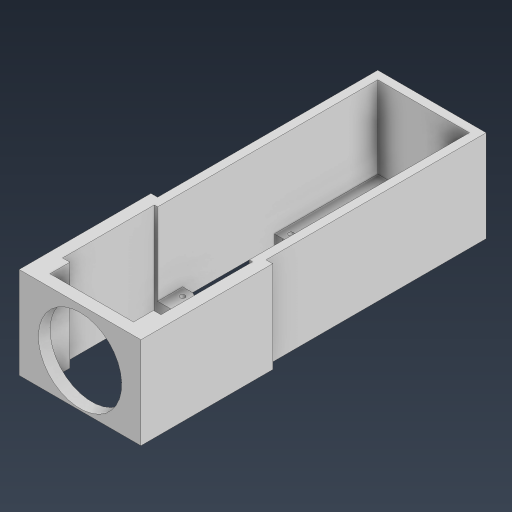
# Autodesk Inventor part: New_base_v2
Saved by Autodesk Inventor 2024 (Build 280153000, 153)
## iProperties
Created: 2025-10-20
Part Number: New_base_v2
Material: Generic
Document SubType Name: Modeling
Designer: Piter
Density: 1 g/cm^3
Appearance: Default
Author: Piter
Autodesk Inventor part; units mm, degrees
ref_plane "YZ Plane" through (0, 0, 0) normal (1, 0, 0) x (0, 1, 0)
ref_plane "XZ Plane" through (0, 0, 0) normal (0, 1, 0) x (-1, 0, 0)
ref_plane "XY Plane" through (0, 0, 0) normal (0, 0, 1) x (1, 0, 0)
sketch "Sketch1" plane through (0, 0, 0) normal (0, 1, 0) x (-1, 0, 0)
  line L0 (-22.5, 32.5) -> (22.5, 32.5) construction
  line L1 (22.5, 32.5) -> (22.5, -32.5) construction
  line L2 (22.5, -32.5) -> (-22.5, -32.5) construction
  line L3 (-22.5, -32.5) -> (-22.5, 32.5) construction
  line L4 (-22.5, 32.5) -> (22.5, -32.5) construction
  line L5 (22.5, 32.5) -> (-22.5, -32.5) construction
  circle A0 centre (22.5, 32.5) radius 1.5
  circle A1 centre (22.5, -32.5) radius 1.5
  circle A2 centre (-22.5, -32.5) radius 1.5
  circle A3 centre (-22.5, 32.5) radius 1.5
  line L6 (27.5, 30) -> (-27.5, 30)
  line L7 (-27.5, 30) -> (-27.5, 37.5)
  line L8 (-27.5, 37.5) -> (27.5, 37.5)
  line L9 (27.5, 37.5) -> (27.5, 30)
  line L10 (27.5, -30) -> (27.5, -37.5)
  line L11 (27.5, -37.5) -> (-27.5, -37.5)
  line L12 (-27.5, -37.5) -> (-27.5, -30)
  line L13 (-27.5, -30) -> (27.5, -30)
  circle A4 centre (22.5, 32.5) radius 5
  circle A5 centre (22.5, -32.5) radius 5
  circle A6 centre (-22.5, -32.5) radius 5
  circle A7 centre (-22.5, 32.5) radius 5
  line L14 (-27.5, 37.5) -> (27.5, 37.5)
  line L15 (27.5, 37.5) -> (27.5, -37.5)
  line L16 (27.5, -37.5) -> (-27.5, -37.5)
  line L17 (-27.5, -37.5) -> (-27.5, 37.5)
  line L18 (-27.5, 37.5) -> (27.5, -37.5) construction
  line L19 (27.5, 37.5) -> (-27.5, -37.5) construction
  line L20 (-32.5, 42.5) -> (32.5, 42.5)
  line L21 (32.5, 42.5) -> (32.5, -42.5)
  line L22 (32.5, -42.5) -> (-32.5, -42.5)
  line L23 (-32.5, -42.5) -> (-32.5, 42.5)
  line L24 (-32.5, 42.5) -> (32.5, -42.5) construction
  line L25 (32.5, 42.5) -> (-32.5, -42.5) construction
  line L26 (32.5, 42.5) -> (-14.872, 42.5)
  line L27 (0, 0) -> (0, -184) construction
  line L28 (-21, -47.5) -> (21, -47.5)
  line L29 (21, -47.5) -> (21, -89.5)
  line L30 (21, -89.5) -> (-21, -89.5)
  line L31 (-21, -89.5) -> (-21, -47.5)
  line L32 (-21, -47.5) -> (21, -89.5) construction
  line L33 (21, -47.5) -> (-21, -89.5) construction
  line L34 (32.5, -42.5) -> (32.5, -94.5)
  line L35 (32.5, -94.5) -> (-32.5, -94.5)
  line L36 (-32.5, -94.5) -> (-32.5, -42.5)
  line L37 (22.5, 27.5) -> (27.5, 27.5)
  line L38 (22.5, -27.5) -> (27.5, -27.5)
  line L39 (-22.5, -27.5) -> (-27.5, -27.5)
  line L40 (-22.5, 27.5) -> (-27.5, 27.5)
  line L41 (0, 0) -> (0, 113) construction
  line L42 (32.5, 42.5) -> (32.5, 97.5)
  line L43 (32.5, 97.5) -> (-32.5, 97.5)
  line L44 (-32.5, 97.5) -> (-32.5, 42.5)
  line L45 (29.5, 42.5) -> (29.5, 97.5)
  line L46 (-29.5, 97.5) -> (-29.5, 42.5)
  line L47 (32.5, 42.5) -> (36.5, 42.5)
  line L48 (36.5, 42.5) -> (36.5, 112.5)
  line L49 (36.5, 112.5) -> (-36.5, 112.5)
  line L50 (-36.5, 112.5) -> (-36.5, 42.5)
  line L51 (-36.5, 42.5) -> (-32.5, 42.5)
  line L52 (-27.5, 37.5) -> (-36.5, 37.5)
  line L53 (-36.5, 37.5) -> (-36.5, 42.5)
  line L54 (-27.5, -27.5) -> (-26.5, -27.5)
  line L55 (-26.5, -27.5) -> (-26.5, 27.5)
  line L56 (0, 112.5) -> (0, 97.5)
  line L57 (-25.05, 112.5) -> (25.05, 112.5)
  line L58 (25.05, 112.5) -> (25.05, 97.5)
  line L59 (25.05, 97.5) -> (-25.05, 97.5)
  line L60 (-25.05, 97.5) -> (-25.05, 112.5)
  line L61 (-25.05, 112.5) -> (25.05, 97.5) construction
  line L62 (25.05, 112.5) -> (-25.05, 97.5) construction
  line L63 (25.05, 109.5) -> (-25.05, 109.5)
  line L64 (36.5, 112.5) -> (-36.5, 112.5)
  line L65 (-36.5, 112.5) -> (-36.5, 116.5)
  line L66 (-36.5, 116.5) -> (36.5, 116.5)
  line L67 (36.5, 116.5) -> (36.5, 112.5)
  line L68 (36.5, 42.5) -> (36.5, 37.5)
  line L69 (36.5, 37.5) -> (32.5, 37.5)
  point P0 (0, -68.5)
  point P1 (18.1699, 30)
  point P2 (18.1699, -30)
  point P3 (-18.1699, -30)
  point P4 (-18.1699, 30)
  point P5 (-32.5, 70)
  point P6 (32.5, 0)
  point P7 (-32.5, 37.5)
  point P8 (0, 105)
  point P9 (-25.05, 97.5)
  dimension "d8" = 10
  dimension "d9" = 10
  dimension "d10" = 10
  dimension "d11" = 10
  dimension "d0" = 45
  dimension "d1" = 65
  dimension "d2" = 3
  dimension "d3" = 3
  dimension "d4" = 3
  dimension "d5" = 3
  dimension "d6" = 2.5
  dimension "d7" = 2.5
  dimension "d12" = 5
  dimension "d13" = 5
  dimension "d17" = 42
  dimension "d18" = 42
  dimension "d19" = 5
  dimension "d20" = 5
  dimension "d38" = 55
  dimension "d39" = 3
  dimension "d40" = 3
  dimension "d41" = 4
  dimension "d42" = 4
  dimension "d43" = 15
  dimension "d57" = 1
  dimension "d72" = 50.1
  dimension "d84" = 7
  dimension "d85" = 3
  constraints: 141 end point, 29 perpendicular, 22 point on line, 15 horizontal, 15 midpoint, 12 parallel, 9 vertical, 8 coincident, 4 centre point, 2 collinear, 12 other
  measures "d0" distance of L1.end L2.end
  measures "d1" distance of L0.end L1.end
  measures "d2" diameter of A0
  measures "d3" diameter of A1
  measures "d4" diameter of A2
  measures "d5" diameter of A3
  measures "d6" distance from line of A0.centre L6
  measures "d7" distance from line of L1.end L13
  measures "d12" distance between parallel lines of L15 L21
  measures "d13" distance between parallel lines of L22 L16
  measures "d17" distance of L29.end L30.end
  measures "d18" distance of L28.end L29.end
  measures "d19" distance between parallel lines of L22 L28
  measures "d20" distance between parallel lines of L30 L35
  measures "d38" distance of L20.end L42.end
  measures "d39" distance from line of point (-32.5, 70) L46
  measures "d40" distance between parallel lines of L42 L45
  measures "d41" distance between parallel lines of L50 L44
  measures "d42" distance between parallel lines of L48 L42
  measures "d43" distance between parallel lines of L49 L43
  measures "d57" distance of L39.end L54.end
  measures "d72" distance of L58.end L59.end
  measures "d84" distance between parallel lines of L66 L63
  measures "d85" distance between parallel lines of L63 L49
extrude "Extrusion1" add sketch "Sketch1" along normal blind 6 contours L15 L37 A4 L6 | L6 A4 L9 | L23 L20 L21 L22 | L52 L53 L51 L23 | A4 L6 | L6 A4 | A4 L8 L9 | L6 A7 L8 A4 | L15 L13 A5 L38 | A7 L6 | L6 A7 | A7 L7 L8 | L10 A5 L13 | A5 L13 | A7 L40 L17 L6 | L6 L7 A7 | A5 L13 | L10 L11 A5 | A5 L11 A6 L13 | A6 L13 | L13 A6 | L39 A6 L13 L17 | L22 L34 L35 L36 | L44 L43 L46 L20 | L51 L50 L49 L60 L43 L44 | L11 L12 A6 | A6 L12 L13 | L21 L47 L68 L69 | L65 L66 L67 L49 | L20 L45 L43 L42 | L42 L43 L58 L49 L48 L47 | L49 L56 L63 L60 | L49 L58 L63 L56 | L28 L29 L30 L31
sketch "Sketch3" plane through (0, 6, 0) normal (0, 1, 0) x (1, 0, 0)
  line L0 (-29.5, -97.5) -> (-29.5, -42.5) projected
  line L1 (-29.5, -42.5) -> (29.5, -42.5) projected
  circle A0 centre (-22.5, -32.5) radius 1.5 projected
  circle A1 centre (22.5, 32.5) radius 1.5 projected
  circle A2 centre (22.5, -32.5) radius 1.5 projected
  circle A3 centre (-22.5, 32.5) radius 1.5 projected
  arc A4 (-18.1699, -30) -> (-22.5, -27.5) centre (-22.5, -32.5) ccw projected
  line L2 (-22.5, -27.5) -> (-27.5, -27.5) projected
  line L3 (-27.5, -27.5) -> (-27.5, 27.5) projected
  line L4 (-27.5, 27.5) -> (-22.5, 27.5) projected
  arc A5 (-22.5, 27.5) -> (-18.1699, 30) centre (-22.5, 32.5) ccw projected
  line L5 (-18.1699, 30) -> (18.1699, 30) projected
  arc A6 (18.1699, 30) -> (22.5, 27.5) centre (22.5, 32.5) ccw projected
  line L6 (22.5, 27.5) -> (27.5, 27.5) projected
  line L7 (27.5, 27.5) -> (27.5, -27.5) projected
  line L8 (27.5, -27.5) -> (22.5, -27.5) projected
  arc A7 (22.5, -27.5) -> (18.1699, -30) centre (22.5, -32.5) ccw projected
  line L9 (18.1699, -30) -> (-18.1699, -30) projected
  line L10 (32.5, -37.5) -> (32.5, 94.5) projected
  line L11 (32.5, 94.5) -> (-32.5, 94.5) projected
  line L12 (-32.5, 94.5) -> (-32.5, -37.5) projected
  line L13 (-29.5, -97.5) -> (-32.5, -97.5)
  line L14 (-29.5, -97.5) -> (-29.5, -42.5) projected
  line L15 (-29.5, -42.5) -> (-32.5, -42.5)
  line L16 (-32.5, -42.5) -> (-32.5, -97.5)
  line L17 (29.5, -97.5) -> (32.5, -97.5)
  line L18 (32.5, -97.5) -> (32.5, -42.5)
  line L19 (32.5, -42.5) -> (29.5, -42.5)
  line L20 (-32.5, 0) -> (-27.5, 0)
  line L21 (-27.5, 27.5) -> (-27.5, 94.5)
  line L22 (27.5, 27.5) -> (27.5, 94.5)
  line L23 (32.5, 94.5) -> (-32.5, 94.5) projected
  line L24 (36.5, -37.5) -> (32.5, -37.5) projected
  line L25 (27.5, -27.5) -> (27.5, -42.5)
  line L26 (32.5, -31.5) -> (27.5, -31.5)
  line L27 (32.5, -2.5) -> (27.5, -2.5)
  line L28 (27.5, -31.5) -> (27.5, -2.5)
  line L29 (27.5, -17) -> (32.5, -17) construction
  line L30 (-25.05, -97.5) -> (-29.5, -97.5) projected
  line L31 (-36.5, -116.5) -> (36.5, -116.5) projected
  line L32 (36.5, -116.5) -> (36.5, -37.5) projected
  line L33 (-32.5, -37.5) -> (-36.5, -37.5) projected
  line L34 (-36.5, -37.5) -> (-36.5, -116.5) projected
  line L35 (29.5, -42.5) -> (29.5, -97.5) projected
  line L36 (29.5, -97.5) -> (25.05, -97.5) projected
  line L37 (25.05, -97.5) -> (25.05, -109.5) projected
  line L38 (25.05, -109.5) -> (-25.05, -109.5) projected
  line L39 (-25.05, -109.5) -> (-25.05, -97.5) projected
  line L40 (-27.5, -27.5) -> (-27.5, -42.5)
  line L41 (27.5, 89.5) -> (-27.5, 89.5)
  point P0 (0, 0)
  point P1 (27.5, 0)
  point P2 (30, -2.5)
  point P3 (30, -31.5)
  point P4 (-32.5, -42.5)
  dimension "d44" = 3
  dimension "d45" = 3
  dimension "d48" = 29
  dimension "d49" = 1
  dimension "d107" = 5
  constraints: 32 end point, 13 point on line, 11 perpendicular, 5 midpoint, 3 horizontal, 1 collinear
  measures "d44" distance between parallel lines of L0 L16
  measures "d45" distance of L17.start L17.end
  measures "d48" distance from line of L26 point (30, -2.5)
  measures "d49" vertical distance of A2.centre point (30, -31.5)
  measures "d107" distance between parallel lines of L23 L41
extrude "Extrusion3" add sketch "Sketch3" along normal blind 45 contours L13 L16 L15 L0 | L30 L39 L38 L37 L36 L17 L18 L19 L1 L25 L26 L10 L24 L32 L31 L34 L33 L12 L20 L3 L40 L15 L16 L13 | L19 L18 L17 L35 | L25 L7 L27 L10 L26 | L20 L12 L11 L21 L3 | L7 L22 L11 L10 L27 | L21 L11 L22 L41
sketch "Sketch7" plane through (25.05, 0, 109.5) normal (0, 0, -1) x (-1, 0, 0)
  line L0 (4.05, 6) -> (46.05, 6) projected
  line L1 (0, 0) -> (50.1, 0) projected
  line L2 (50.1, 0) -> (50.1, 51) projected
  line L3 (0, 0) -> (0, 51) projected
  line L4 (25.05, 51) -> (25.05, 0) construction
  line L5 (5.05, 46) -> (45.05, 46)
  line L6 (45.05, 46) -> (45.05, 6)
  line L7 (45.05, 6) -> (5.05, 6)
  line L8 (5.05, 6) -> (5.05, 46)
  line L9 (5.05, 46) -> (45.05, 6) construction
  line L10 (45.05, 46) -> (5.05, 6) construction
  circle A0 centre (45.05, 6) radius 2
  circle A1 centre (45.05, 46) radius 2
  circle A2 centre (5.05, 46) radius 2
  circle A3 centre (5.05, 6) radius 2
  circle A4 centre (25.05, 26) radius 25
  line L11 (0, 51) -> (50.1, 51) projected
  dimension "d74" = 40
  dimension "d75" = 40
  dimension "d77" = 4
  dimension "d78" = 4
  dimension "d79" = 4
  dimension "d80" = 4
  dimension "d81" = 50
  dimension "d86" = 6
  constraints: 14 end point, 5 centre point, 5 coincident, 2 midpoint, 2 parallel, 1 horizontal, 1 perpendicular, 1 point on line
  measures "d74" distance of L6.end L7.end
  measures "d75" distance of L5.end L6.end
  measures "d77" diameter of A0
  measures "d78" diameter of A1
  measures "d79" diameter of A2
  measures "d80" diameter of A3
  measures "d81" diameter of A4
  measures "d86" distance between parallel lines of L1 L7
extrude "Extrusion9" cut sketch "Sketch7" against normal blind 45 contours A4 L8 L5 L6 L0 | L0 A4 | A4 L8 | L6 A4 | A4 L5
extrude "Extrusion10" cut sketch "Sketch7" against normal blind 5 contours L8 A3 L0 | L0 A3 L8 | A0 L6 L0 | L0 L6 A0 | A2 L5 L8 | L8 L5 A2 | A1 L5 L6 | L6 L5 A1
sketch "Sketch8" plane through (0, 51, 0) normal (0, 1, 0) x (1, 0, 0)
  line L0 (32.5, 94.5) -> (-32.5, 94.5) projected
  line L1 (-32.5, 94.5) -> (-32.5, -37.5) projected
  line L2 (-36.5, -116.5) -> (0, -116.5) projected
  line L3 (36.5, -116.5) -> (36.5, -37.5) projected
  line L4 (36.5, -37.5) -> (32.5, -37.5) projected
  line L5 (32.5, -37.5) -> (32.5, 94.5) projected
  line L6 (-36.5, -42.5) -> (36.5, -42.5)
  line L7 (-32.5, -37.5) -> (-36.5, -37.5) projected
  line L8 (-36.5, -37.5) -> (-36.5, -116.5) projected
  line L9 (0, -109.5) -> (0, -116.5) projected
  line L10 (0, -116.5) -> (36.5, -116.5) projected
  line L11 (27.5, -42.5) -> (29.5, -42.5) projected
  line L12 (29.5, -42.5) -> (29.5, -97.5) projected
  line L13 (29.5, -97.5) -> (25.05, -97.5) projected
  line L14 (25.05, -97.5) -> (25.05, -109.5) projected
  line L15 (25.05, -109.5) -> (0, -109.5) projected
  line L16 (0, -109.5) -> (-25.05, -109.5) projected
  line L17 (-25.05, -109.5) -> (-25.05, -97.5) projected
  line L18 (-25.05, -97.5) -> (-29.5, -97.5) projected
  line L19 (-29.5, -97.5) -> (-29.5, -42.5) projected
  line L20 (27.5, 89.5) -> (27.5, -42.5) projected
  line L21 (-29.5, -42.5) -> (-27.5, -42.5) projected
  line L22 (-27.5, -42.5) -> (-27.5, 89.5) projected
  line L23 (-27.5, 89.5) -> (27.5, 89.5) projected
  point P0 (0, 0)
  constraints: 2 end point, 1 perpendicular, 1 point on line
extrude "Extrusion11" add sketch "Sketch8" along normal blind 4 contours L5 L4 L3 L6 L20 L23 L22 L8 L7 L1 L0 | L3 L10 L9 L15 L14 L13 L12 L6 | L6 L19 L18 L17 L16 L9 L2 L8
body "Solid1"
